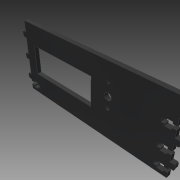
# Autodesk Inventor part: front_panel_2004_display
Saved by Autodesk Inventor 2014 (Build 180170000, 170)
## iProperties
Created: 2014-01-11
Part Number: front_panel_2004_display
Material: Generic
Document SubType Name: Modeling
Designer: buben
Density: 1 g/cm^3
Appearance: Anodized - Dark Gray
Author: buben
Autodesk Inventor part; units mm, degrees
ref_plane "YZ Plane" through (0, 0, 0) normal (1, 0, 0) x (0, 1, 0)
ref_plane "XZ Plane" through (0, 0, 0) normal (0, 1, 0) x (-1, 0, 0)
ref_plane "XY Plane" through (0, 0, 0) normal (0, 0, 1) x (1, 0, 0)
sketch "Sketch1" plane through (0, 0, 0) normal (0, 1, 0) x (-1, 0, 0)
  line L0 (0, 0) -> (220, 0)
  line L1 (220, 0) -> (220, 100)
  line L2 (220, 100) -> (0, 100)
  line L3 (0, 100) -> (0, 0)
  dimension "d11" = 220
  dimension "d16" = 100
  constraints: 8 end point, 2 parallel, 1 horizontal, 1 perpendicular
  measures "d11" distance of L0.start L0.end
  measures "d16" distance of L2.end L0.start
extrude "Extrusion3" add sketch "Sketch1" along normal blind 6
sketch "Sketch3" plane through (0, 0, 0) normal (0, -1, 0) x (1, 0, 0)
  line L0 (0, 100) -> (0, 0) projected
  line L1 (-220, 0) -> (-220, 100) projected
  line L2 (-220, 85) -> (-224, 85)
  line L3 (-226, 83) -> (-226, 79)
  line L4 (-224, 77) -> (-220, 77)
  line L5 (-220, 77) -> (-220, 85)
  line L6 (-220, 54) -> (-224, 54)
  line L7 (-226, 52) -> (-226, 48)
  line L8 (-224, 46) -> (-220, 46)
  line L9 (-220, 46) -> (-220, 54)
  line L10 (-220, 23) -> (-224, 23)
  line L11 (-226, 21) -> (-226, 17)
  line L12 (-224, 15) -> (-220, 15)
  line L13 (-220, 15) -> (-220, 23)
  line L14 (0, 85) -> (4, 85)
  line L15 (6, 83) -> (6, 79)
  line L16 (4, 77) -> (0, 77)
  line L17 (0, 77) -> (0, 85)
  line L18 (0, 54) -> (4, 54)
  line L19 (6, 52) -> (6, 48)
  line L20 (4, 46) -> (0, 46)
  line L21 (0, 46) -> (0, 54)
  line L22 (0, 23) -> (4, 23)
  line L23 (6, 21) -> (6, 17)
  line L24 (4, 15) -> (0, 15)
  line L25 (0, 15) -> (0, 23)
  arc A0 (-224, 85) -> (-226, 83) centre (-224, 83) ccw
  arc A1 (-226, 79) -> (-224, 77) centre (-224, 79) ccw
  arc A2 (-224, 54) -> (-226, 52) centre (-224, 52) ccw
  arc A3 (-226, 48) -> (-224, 46) centre (-224, 48) ccw
  arc A4 (-224, 23) -> (-226, 21) centre (-224, 21) ccw
  arc A5 (-226, 17) -> (-224, 15) centre (-224, 17) ccw
  arc A6 (6, 83) -> (4, 85) centre (4, 83) ccw
  arc A7 (4, 77) -> (6, 79) centre (4, 79) ccw
  arc A8 (6, 52) -> (4, 54) centre (4, 52) ccw
  arc A9 (4, 46) -> (6, 48) centre (4, 48) ccw
  arc A10 (6, 21) -> (4, 23) centre (4, 21) ccw
  arc A11 (4, 15) -> (6, 17) centre (4, 17) ccw
  line L26 (-222, 77) -> (-222, 54) construction
  line L27 (-222, 23) -> (-222, 46) construction
  point P0 (-226, 50)
  point P1 (-220, 50)
  dimension "d35" = 2
  dimension "d36" = 8
  dimension "d37" = 6
  dimension "d38" = 8
  dimension "d39" = 8
  dimension "d40" = 8
  dimension "d41" = 8
  dimension "d42" = 8
  dimension "d43" = 6
  dimension "d44" = 23
  constraints: 52 end point, 24 point on circle, 24 tangent, 12 centre point, 12 parallel, 11 equal radius, 8 collinear, 6 horizontal, 6 midpoint, 6 perpendicular, 6 point on line, 1 horizontal alignment
  measures "d35" radius of A0
  measures "d36" distance between parallel lines of L4 L2
  measures "d37" distance between parallel lines of L5 L3
  measures "d38" distance between parallel lines of L8 L6
  measures "d39" distance between parallel lines of L12 L10
  measures "d40" distance between parallel lines of L16 L14
  measures "d41" distance between parallel lines of L20 L18
  measures "d42" distance between parallel lines of L24 L22
  measures "d43" distance from line of L0 L15.end
  measures "d44" distance of L26.start L26.end
extrude "Extrusion4" add sketch "Sketch3" against normal blind 6
sketch "Sketch4" plane through (0, 0, 0) normal (0, -1, 0) x (1, 0, 0)
  line L0 (-220, 100) -> (0, 100) projected
  line L1 (-220, 54) -> (-220, 77) projected
  line L2 (-204, 71) -> (-106, 71) construction
  line L3 (-106, 71) -> (-106, 31) construction
  line L4 (-106, 31) -> (-204, 31) construction
  line L5 (-204, 31) -> (-204, 71) construction
  line L6 (-204.5, 71.5) -> (-105.5, 71.5)
  line L7 (-105.5, 71.5) -> (-105.5, 30.5)
  line L8 (-105.5, 30.5) -> (-204.5, 30.5)
  line L9 (-204.5, 30.5) -> (-204.5, 71.5)
  circle A0 centre (-81, 75) radius 1.5
  circle A1 centre (-81, 57.5) radius 5
  circle A2 centre (-81, 42) radius 2.5
  line L10 (-218, 85) -> (-68, 85) construction
  line L11 (-68, 85) -> (-68, 30) construction
  line L12 (-68, 30) -> (-218, 30) construction
  line L13 (-218, 30) -> (-218, 85) construction
  point P0 (-155, 71.5)
  point P1 (-155, 71)
  point P2 (-106, 51)
  point P3 (-105.5, 51)
  dimension "d47" = 40
  dimension "d48" = 98
  dimension "d49" = 99
  dimension "d50" = 41
  dimension "d51" = 25
  dimension "d52" = 5
  dimension "d53" = 15.5
  dimension "d54" = 17.5
  dimension "d55" = 13.5
  dimension "d56" = 3
  dimension "d57" = 10
  dimension "d58" = 55
  dimension "d59" = 150
  dimension "d60" = 14
  dimension "d61" = 14
  dimension "d62" = 15
  dimension "d63" = 2
  constraints: 24 end point, 6 parallel, 4 midpoint, 3 centre point, 3 horizontal, 3 perpendicular, 3 vertical alignment, 1 horizontal alignment
  measures "d47" distance of L2.end L3.end
  measures "d48" distance of L3.end L4.end
  measures "d49" distance of L7.end L8.end
  measures "d50" distance of L6.end L7.end
  measures "d51" distance from line of A1.centre L3
  measures "d52" diameter of A2
  measures "d53" distance of A2.centre A1.centre
  measures "d54" distance of A0.centre A1.centre
  measures "d55" distance from line of A1.centre L2
  measures "d56" diameter of A0
  measures "d57" diameter of A1
  measures "d58" distance of L12.end L10.start
  measures "d59" distance of L10.start L10.end
  measures "d60" distance between parallel lines of L5 L13
  measures "d61" distance between parallel lines of L10 L2
  measures "d62" distance between parallel lines of L0 L10
  measures "d63" distance between parallel lines of L1 L13
extrude "Extrusion5" cut sketch "Sketch4" against normal through all
sketch "Sketch5" plane through (0, 0, 0) normal (0, -1, 0) x (1, 0, 0)
  line L0 (0, 0) -> (-220, 0) projected
  line L1 (0, 46) -> (0, 23) projected
  line L2 (0, 77) -> (0, 54) projected
  line L3 (-220, 100) -> (0, 100) projected
  line L4 (-220, 0) -> (-220, 15) projected
  line L5 (-203.7, 12) -> (-203.7, 7.5)
  line L6 (-220, 7.5) -> (-220, 12)
  line L7 (-215, 14.5) -> (-207.7, 14.5)
  line L8 (-207.7, 5) -> (-215, 5)
  line L9 (-220, 12) -> (-215, 12)
  line L10 (-207.7, 12) -> (-203.7, 12)
  line L11 (-203.7, 7.5) -> (-207.7, 7.5)
  line L12 (-215, 7.5) -> (-220, 7.5)
  line L13 (-215, 5) -> (-215, 7.5)
  line L14 (-215, 12) -> (-215, 14.5)
  line L15 (-207.7, 14.5) -> (-207.7, 12)
  line L16 (-207.7, 7.5) -> (-207.7, 5)
  line L17 (-110, 100) -> (-110, -1.0971) construction
  line L18 (-16.3, 12) -> (-16.3, 7.5)
  line L19 (0, 7.5) -> (0, 12)
  line L20 (-5, 14.5) -> (-12.3, 14.5)
  line L21 (-12.3, 5) -> (-5, 5)
  line L22 (0, 12) -> (-5, 12)
  line L23 (-12.3, 12) -> (-16.3, 12)
  line L24 (-16.3, 7.5) -> (-12.3, 7.5)
  line L25 (-5, 7.5) -> (0, 7.5)
  line L26 (-5, 5) -> (-5, 7.5)
  line L27 (-5, 12) -> (-5, 14.5)
  line L28 (-12.3, 14.5) -> (-12.3, 12)
  line L29 (-12.3, 7.5) -> (-12.3, 5)
  line L30 (0, 67.75) -> (0, 63.25)
  line L31 (-16.3, 63.25) -> (-16.3, 67.75)
  line L32 (-12.3, 70.25) -> (-5, 70.25)
  line L33 (-5, 60.75) -> (-12.3, 60.75)
  line L34 (-16.3, 67.75) -> (-12.3, 67.75)
  line L35 (-5, 67.75) -> (0, 67.75)
  line L36 (0, 63.25) -> (-5, 63.25)
  line L37 (-12.3, 63.25) -> (-16.3, 63.25)
  line L38 (-12.3, 60.75) -> (-12.3, 63.25)
  line L39 (-12.3, 67.75) -> (-12.3, 70.25)
  line L40 (-5, 70.25) -> (-5, 67.75)
  line L41 (-5, 63.25) -> (-5, 60.75)
  line L42 (0, 36.75) -> (0, 32.25)
  line L43 (-16.3, 32.25) -> (-16.3, 36.75)
  line L44 (-12.3, 39.25) -> (-5, 39.25)
  line L45 (-5, 29.75) -> (-12.3, 29.75)
  line L46 (-16.3, 36.75) -> (-12.3, 36.75)
  line L47 (-5, 36.75) -> (0, 36.75)
  line L48 (0, 32.25) -> (-5, 32.25)
  line L49 (-12.3, 32.25) -> (-16.3, 32.25)
  line L50 (-12.3, 29.75) -> (-12.3, 32.25)
  line L51 (-12.3, 36.75) -> (-12.3, 39.25)
  line L52 (-5, 39.25) -> (-5, 36.75)
  line L53 (-5, 32.25) -> (-5, 29.75)
  point P0 (-203.7, 9.75)
  point P1 (-16.3, 9.75)
  point P2 (0, 65.5)
  point P3 (0, 34.5)
  dimension "d66" = 2.5
  dimension "d67" = 2.5
  dimension "d68" = 5
  dimension "d69" = 4
  dimension "d70" = 7.3
  dimension "d71" = 4.5
  dimension "d72" = 5
  dimension "d73" = 2.5
  dimension "d74" = 2.5
  dimension "d75" = 4
  dimension "d76" = 5
  dimension "d77" = 7.3
  dimension "d78" = 4.5
  dimension "d79" = 2.5
  dimension "d80" = 2.5
  dimension "d81" = 4
  dimension "d82" = 5
  dimension "d83" = 7.3
  dimension "d84" = 4.5
  constraints: 98 end point, 30 parallel, 13 collinear, 13 perpendicular, 13 symmetric about line, 9 horizontal, 6 midpoint
  measures "d66" distance of L11.end L8.start
  measures "d67" distance of L7.end L10.start
  measures "d68" distance of L6.end L9.end
  measures "d69" distance of L10.start L5.start
  measures "d70" distance of L7.start L7.end
  measures "d71" distance of L5.start L5.end
  measures "d72" distance between parallel lines of L0 L8
  measures "d73" distance of L36.end L33.start
  measures "d74" distance of L40.start L35.start
  measures "d75" distance of L34.start L39.start
  measures "d76" distance of L35.start L30.start
  measures "d77" distance of L39.end L40.start
  measures "d78" distance of L30.start L30.end
  measures "d79" distance of L48.end L45.start
  measures "d80" distance of L52.start L47.start
  measures "d81" distance of L46.start L51.start
  measures "d82" distance of L47.start L42.start
  measures "d83" distance of L51.end L52.start
  measures "d84" distance of L42.start L42.end
extrude "Extrusion6" cut sketch "Sketch5" against normal through all
equation "\"d38\" = d36"
equation "\"d39\" = d38"
equation "\"d40\" = d36"
equation "\"d41\" = d40"
equation "\"d42\" = d41"
equation "\"d43\" = d37"
equation "\"d67\" = d66"
equation "\"d74\" = d73"
equation "\"d80\" = d79"
body "Solid2"
